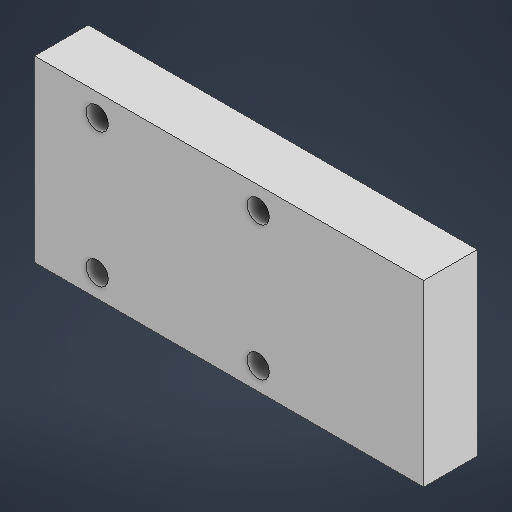
# Autodesk Inventor part: SAFRS-P-0032
Saved by Autodesk Inventor 2026.2 (Build 302298000, 298)
## iProperties
Created: 2025-11-26
Part Number: SAFRS-P-0032
Material: 일반
Document SubType Name: Modeling
Designer: jaewook
Density: 1 g/cm^3
Appearance: 기본값
Author: jaewook
Title: DC Converter
Autodesk Inventor part; units mm, degrees
ref_plane "YZ Plane" through (0, 0, 0) normal (1, 0, 0) x (0, 1, 0)
ref_plane "XZ Plane" through (0, 0, 0) normal (0, 1, 0) x (-1, 0, 0)
ref_plane "XY Plane" through (0, 0, 0) normal (0, 0, 1) x (1, 0, 0)
sketch "스케치1" plane through (0, 0, 0) normal (0, 0, 1) x (1, 0, 0)
  line L0 (-21.75, -10) -> (21.75, -10)
  line L1 (21.75, -10) -> (21.75, 10)
  line L2 (21.75, 10) -> (-21.75, 10)
  line L3 (-21.75, 10) -> (-21.75, -10)
  line L4 (-21.75, -10) -> (21.75, 10) construction
  line L5 (21.75, -10) -> (-21.75, 10) construction
  circle A0 centre (-14.75, -7.5) radius 1.25
  circle A1 centre (3.25, -7.5) radius 1.25
  circle A2 centre (-14.75, 7.5) radius 1.25
  circle A3 centre (3.25, 7.5) radius 1.25
  point P0 (0, 0)
  dimension "d0" = 43.5
  dimension "d1" = 20
  dimension "d4" = 2.5
  dimension "d5" = 2.5
  dimension "d6" = 7
  dimension "d9" = 18
  dimension "d12" = 15
  constraints: 12 end point, 4 centre point, 2 horizontal, 2 midpoint, 2 parallel, 1 perpendicular, 1 vertical, 6 other
  measures "d0" distance of L2.end L1.end
  measures "d1" distance of L1.end L0.end
  measures "d4" diameter of A0
  measures "d5" distance from line of L0 A0.centre
  measures "d6" distance from line of L3 A0.centre
  measures "d9" distance of A0.centre A1.centre
  measures "d12" distance of A0.centre A2.centre
extrude "돌출1" add sketch "스케치1" along normal blind 6
